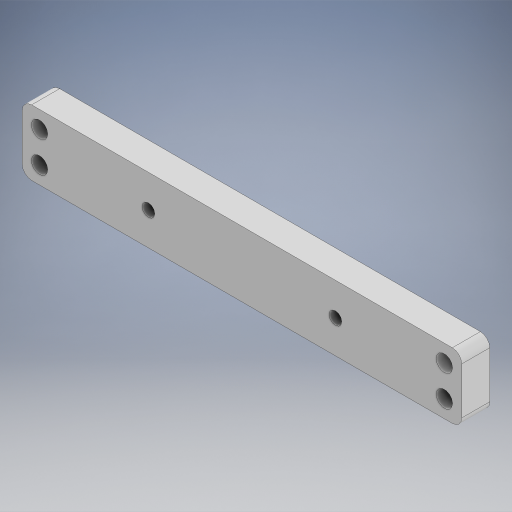
# Autodesk Inventor part: front of head(top)_zig7
Saved by Autodesk Inventor 2024 (Build 280153000, 153)
## iProperties
Created: 2024-09-11
Part Number: front of head(top)_zig7
Material: 일반
Document SubType Name: Modeling
Designer: ASUS
Density: 1 g/cm^3
Appearance: 기본값
Author: ASUS
Autodesk Inventor part; units mm, degrees
ref_plane "YZ Plane" through (0, 0, 0) normal (1, 0, 0) x (0, 1, 0)
ref_plane "XZ Plane" through (0, 0, 0) normal (0, 1, 0) x (-1, 0, 0)
ref_plane "XY Plane" through (0, 0, 0) normal (0, 0, 1) x (1, 0, 0)
ref_plane "작업 평면1" through (0, 0, 0) normal (0, 0, 1) x (1, 0, 0)
sketch "스케치1" plane through (0, 0, 0) normal (0, 0, 1) x (1, 0, 0)
  circle A0 centre (-20, 0) radius 1.35 projected
  line L0 (-6.05, -3) -> (-6.05, 3) projected
  line L1 (-6.05, 3) -> (-43, 3) projected
  line L2 (-43, -3) -> (-43, 3) projected
  line L3 (-6.05, -3) -> (-43, -3) projected
  line L4 (6.05, 3) -> (6.05, -3) projected
  line L5 (6.05, -3) -> (43, -3) projected
  line L6 (43, 3) -> (43, -3) projected
  line L7 (6.05, 3) -> (43, 3) projected
  circle A1 centre (20, 0) radius 1.35 projected
  line L8 (-43, 3) -> (43, 3)
  line L9 (43, 3) -> (43, -3)
  line L10 (43, -3) -> (-43, -3)
  line L11 (-43, -3) -> (-43, 3)
  line L12 (43.3, 3.3) -> (-43.3, 3.3)
  line L13 (-43.3, 3.3) -> (-43.3, -3.3)
  line L14 (-43.3, -3.3) -> (43.3, -3.3)
  line L15 (43.3, -3.3) -> (43.3, 3.3)
  line L16 (47, 7) -> (-47, 7)
  line L17 (-47, 7) -> (-47, -7)
  line L18 (-47, -7) -> (47, -7)
  line L19 (47, -7) -> (47, 7)
  point P0 (0, 0)
  dimension "d0" = 0.3
  dimension "d1" = 4
  constraints: 24 end point, 6 parallel, 3 perpendicular, 1 horizontal, 6 other
  measures "d0" distance between parallel lines of L8 L12
  measures "d1" distance between parallel lines of L8 L16
extrude "돌출1" add sketch "스케치1" along normal blind 3 contours L19 L18 L17 L16
sketch "스케치2" plane through (0, 0, 3) normal (0, 0, 1) x (1, 0, 0)
  line L0 (-47, 7) -> (-47, -7) projected
  line L1 (-47, -7) -> (47, -7) projected
  line L2 (47, -7) -> (47, 7) projected
  line L3 (47, 7) -> (-47, 7) projected
  line L4 (43.3, 3.3) -> (43.3, -3.3) projected
  line L5 (43.3, -3.3) -> (-43.3, -3.3) projected
  line L6 (-43.3, -3.3) -> (-43.3, 3.3) projected
  line L7 (-43.3, 3.3) -> (43.3, 3.3) projected
  circle A0 centre (-20, 0) radius 1.35 projected
  line L8 (-6.05, -3) -> (-6.05, 3) projected
  line L9 (-6.05, 3) -> (-43, 3) projected
  line L10 (-43, -3) -> (-43, 3) projected
  line L11 (-6.05, -3) -> (-43, -3) projected
  line L12 (15, 3) -> (15, -3)
  line L13 (6.05, 3) -> (6.05, -3) projected
  line L14 (6.05, -3) -> (43, -3) projected
  line L15 (43, 3) -> (43, -3) projected
  line L16 (6.05, 3) -> (43, 3) projected
  circle A1 centre (20, 0) radius 1.35 projected
  point P0 (0, 0)
  constraints: 2 end point, 1 vertical, 2 other
extrude "돌출2" add sketch "스케치2" along normal blind 3 contours L3 L2 L1 L0 | L4 L5 L6 L7 | L11 L10 L9 L8 | L16 L15 L14 L12 | L12 L14 L13 L16
sketch "스케치3" plane through (0, 0, 0) normal (0, 0, -1) x (-1, 0, 0)
  line L0 (47, 7) -> (47, -7) projected
  line L1 (-47, 7) -> (47, 7) projected
  line L2 (-47, -7) -> (-47, 7) projected
  line L3 (47, -7) -> (-47, -7) projected
  line L4 (-43.3, 3.3) -> (-43.3, -3.3) projected
  line L5 (43.3, 3.3) -> (-43.3, 3.3) projected
  line L6 (43.3, -3.3) -> (43.3, 3.3) projected
  line L7 (-43.3, -3.3) -> (43.3, -3.3) projected
  point P0 (0, 0)
hole "구멍1" at (43.3, 3.3, 0) at (43.3, -3.3, 0) at (-43.3, 3.3, 0) at (-43.3, -3.3, 0) direction (0, 0, 1) diameter 3.2 end through all
fillet "모깎기1" radius 2 4 edges at (47, 7, 3) (47, -7, 3) (-47, 7, 3) (-47, -7, 3)
sketch "스케치4" plane through (0, 0, 0) normal (0, 0, -1) x (-1, 0, 0)
  arc A0 (45, -7) -> (47, -5) centre (45, -5) ccw projected
  line L0 (47, 5) -> (47, -5) projected
  arc A1 (47, 5) -> (45, 7) centre (45, 5) ccw projected
  line L1 (-45, 7) -> (45, 7) projected
  arc A2 (-45, 7) -> (-47, 5) centre (-45, 5) ccw projected
  line L2 (-47, -5) -> (-47, 5) projected
  arc A3 (-47, -5) -> (-45, -7) centre (-45, -5) ccw projected
  line L3 (45, -7) -> (-45, -7) projected
  arc A4 (41.7, -3.3) -> (43.3, -1.7) centre (43.3, -3.3) ccw projected
  line L4 (-41.7, -3.3) -> (41.7, -3.3) projected
  arc A5 (-43.3, -1.7) -> (-41.7, -3.3) centre (-43.3, -3.3) ccw projected
  line L5 (-43.3, 1.7) -> (-43.3, -1.7) projected
  arc A6 (-41.7, 3.3) -> (-43.3, 1.7) centre (-43.3, 3.3) ccw projected
  line L6 (41.7, 3.3) -> (-41.7, 3.3) projected
  arc A7 (43.3, 1.7) -> (41.7, 3.3) centre (43.3, 3.3) ccw projected
  line L7 (43.3, -1.7) -> (43.3, 1.7) projected
  arc A8 (43.3, -1.7) -> (41.7, -3.3) centre (43.3, -3.3) ccw projected
  line L8 (43.3, -1.7) -> (43.3, 1.7) projected
  arc A9 (41.7, 3.3) -> (43.3, 1.7) centre (43.3, 3.3) ccw projected
  line L9 (41.7, 3.3) -> (-41.7, 3.3) projected
  arc A10 (-43.3, 1.7) -> (-41.7, 3.3) centre (-43.3, 3.3) ccw projected
  line L10 (-43.3, 1.7) -> (-43.3, -1.7) projected
  arc A11 (-41.7, -3.3) -> (-43.3, -1.7) centre (-43.3, -3.3) ccw projected
  line L11 (-41.7, -3.3) -> (41.7, -3.3) projected
  circle A12 centre (20, 0) radius 1.35 projected
  circle A13 centre (-20, 0) radius 1.35 projected
  line L12 (-43.1, 1.9144) -> (-43.1, -1.9144)
  arc A14 (-43.1, -1.9144) -> (-41.9144, -3.1) centre (-43.3, -3.3) ccw
  line L13 (-41.9144, -3.1) -> (41.9144, -3.1)
  arc A15 (41.9144, -3.1) -> (43.1, -1.9144) centre (43.3, -3.3) ccw
  line L14 (43.1, -1.9144) -> (43.1, 1.9144)
  arc A16 (43.1, 1.9144) -> (41.9144, 3.1) centre (43.3, 3.3) ccw
  line L15 (41.9144, 3.1) -> (-41.9144, 3.1)
  arc A17 (-41.9144, 3.1) -> (-43.1, 1.9144) centre (-43.3, 3.3) ccw
  point P0 (0, 0)
  point P1 (41.7125, -3.1)
  point P2 (-41.7125, -3.1)
  point P3 (-43.1, -1.7125)
  point P4 (-43.1, 1.7125)
  point P5 (-41.7125, 3.1)
  point P6 (41.7125, 3.1)
  point P7 (43.1, 1.7125)
  point P8 (43.1, -1.7125)
  dimension "d14" = 0.2
  constraints: 8 end point, 8 point on circle, 4 centre point, 7 other
  measures "d14" radial gap between concentric circles of A6 A17
extrude "돌출3" add sketch "스케치4" against normal up to surface (6 mm away) contours A8 L13 A15 L14 A4 | L4 A11 L13 A8 | A8 L14 A9 L7 | A5 A11 L12 A14 L13 | A9 L14 A16 L15 A7 | L5 A10 L12 A11 | A9 L15 A10 L6 | A6 A10 L15 A17 L12
sketch "스케치5" plane through (0, 0, 0) normal (0, 0, -1) x (-1, 0, 0)
  line L0 (41.9144, -3.1) -> (-41.9144, -3.1) projected
  arc A0 (-43.1, -1.9144) -> (-41.9144, -3.1) centre (-43.3, -3.3) ccw projected
  line L1 (-43.1, -1.9144) -> (-43.1, 1.9144) projected
  arc A1 (-41.9144, 3.1) -> (-43.1, 1.9144) centre (-43.3, 3.3) ccw projected
  line L2 (-41.9144, 3.1) -> (41.9144, 3.1) projected
  arc A2 (43.1, 1.9144) -> (41.9144, 3.1) centre (43.3, 3.3) ccw projected
  line L3 (43.1, 1.9144) -> (43.1, -1.9144) projected
  arc A3 (41.9144, -3.1) -> (43.1, -1.9144) centre (43.3, -3.3) ccw projected
  arc A4 (45, -7) -> (47, -5) centre (45, -5) ccw projected
  line L4 (47, 5) -> (47, -5) projected
  arc A5 (47, 5) -> (45, 7) centre (45, 5) ccw projected
  line L5 (-45, 7) -> (45, 7) projected
  arc A6 (-45, 7) -> (-47, 5) centre (-45, 5) ccw projected
  line L6 (-47, -5) -> (-47, 5) projected
  arc A7 (-47, -5) -> (-45, -7) centre (-45, -5) ccw projected
  line L7 (45, -7) -> (-45, -7) projected
  point P0 (0, 0)
hole "구멍2" at (-43.3, -3.3, 0) at (-43.3, 3.3, 0) at (43.3, -3.3, 0) at (43.3, 3.3, 0) direction (0, 0, 1) diameter 3.5 end through all
